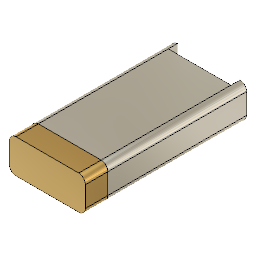
kneelingpad_fusion v6 (Autodesk Fusion 360 archive; units mm, degrees)
design "3898 400mAh Battery"
Autodesk Fusion 360 part; units mm, degrees
sketch "Sketch1" plane through (0, 0, 0) normal (0, 0, 1) x (1, 0, 0)
  line L0 (0, 0) -> (17, 0)
  line L1 (17, 0) -> (17, 36)
  line L2 (17, 36) -> (0, 36)
  line L3 (0, 36) -> (0, 0)
  line L4 (15.5, 34) -> (1.5, 34)
  line L5 (1.5, 34) -> (1.5, 36)
  line L6 (1.5, 36) -> (15.5, 36)
  line L7 (15.5, 36) -> (15.5, 34)
  dimension "d1" = 17
  dimension "d2" = 36
  dimension "d7" = 2
  dimension "d8" = 14
  measures "d1" distance of L0.start
  measures "d2" distance of L0.start
extrude "Extrude1" add sketch "Sketch1" along normal blind 7.6 contours L0 L1 L2 L3 L4 L5 L7 makes body 1
ref_plane "WorkPlane1" through (8.5, 5, 3.8) normal (0, -1, 0) x (1, 0, 0)
fillet "Fillet1" radius 1.5 4 edges at (17, 18, 7.6) (17, 18, 0) (0, 18, 7.6) (0, 18, 0) on bodies 1
split "Split1" by plane through (8.5, 5, 3.8) normal (0, -1, 0) bodies 1 makes body 2 at (10.8334, 0, 5.0667)
